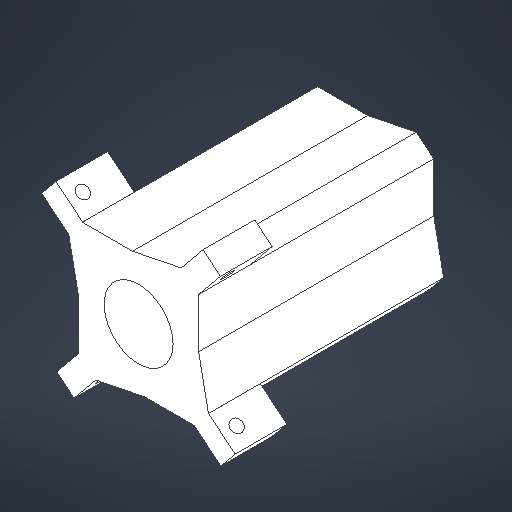
# Autodesk Inventor part: Lifter compartment
Saved by Autodesk Inventor 2026.1 (Build 301233020, 233B)
## iProperties
Created: 2025-11-27
Part Number: Lifter compartment
Material: Generic
Document SubType Name: Modeling
Designer: sarab
Density: 1 g/cm^3
Appearance: Default
Author: sarab
Autodesk Inventor part; units mm, degrees
ref_plane "YZ Plane" through (0, 0, 0) normal (1, 0, 0) x (0, 1, 0)
ref_plane "XZ Plane" through (0, 0, 0) normal (0, 1, 0) x (-1, 0, 0)
ref_plane "XY Plane" through (0, 0, 0) normal (0, 0, 1) x (1, 0, 0)
sketch "Sketch1" plane through (0, 0, 0) normal (0, 0, 1) x (1, 0, 0)
  circle A0 centre (-38.3507, 10.1677) radius 10.4
  line L0 (-51.23, -10.8726) -> (-51.1921, -10.9035)
  line L1 (-51.1921, -10.9035) -> (-36.539, -7.9419)
  line L2 (-36.539, -7.9419) -> (-21.5895, -7.9419)
  line L3 (-21.5895, -7.9419) -> (-13.5401, -14.5272)
  line L4 (-9.2136, -9.2389) -> (-13.5401, -14.5272)
  line L5 (-17.2631, -2.6536) -> (-9.2136, -9.2389)
  line L6 (-17.2631, -2.6536) -> (-17.2795, -2.6737)
  line L7 (-17.2795, -2.6737) -> (-20.2411, 11.9795)
  line L8 (-20.2411, 11.9795) -> (-20.2411, 26.9289)
  line L9 (-20.2411, 26.9289) -> (-13.6558, 34.9784)
  line L10 (-18.9241, 39.2883) -> (-13.6558, 34.9784)
  line L11 (-25.5094, 31.2389) -> (-18.9241, 39.2883)
  line L12 (-25.5094, 31.2389) -> (-40.1625, 28.2773)
  line L13 (-40.1625, 28.2773) -> (-55.3133, 28.2773)
  line L14 (-55.3133, 28.2773) -> (-55.2326, 28.3759)
  line L15 (-55.2326, 28.3759) -> (-63.282, 34.9612)
  line L16 (-67.592, 29.693) -> (-63.282, 34.9612)
  line L17 (-59.5426, 23.1077) -> (-67.592, 29.693)
  line L18 (-59.5426, 23.1077) -> (-59.4618, 23.2064)
  line L19 (-59.4618, 23.2064) -> (-56.4603, 8.3559)
  line L20 (-56.4603, 8.3559) -> (-56.4603, -6.5936)
  line L21 (-56.4603, -6.5936) -> (-63.0456, -14.643)
  line L22 (-57.8153, -18.922) -> (-63.0456, -14.643)
  line L23 (-51.23, -10.8726) -> (-57.8153, -18.922)
  circle A1 centre (-38.3507, 10.1677) radius 10.4
  line L24 (-51.23, -10.8726) -> (-51.1921, -10.9035)
  line L25 (-51.1921, -10.9035) -> (-36.539, -7.9419)
  line L26 (-36.539, -7.9419) -> (-21.5895, -7.9419)
  line L27 (-21.5895, -7.9419) -> (-13.5401, -14.5272)
  line L28 (-9.2136, -9.2389) -> (-13.5401, -14.5272)
  line L29 (-17.2631, -2.6536) -> (-9.2136, -9.2389)
  line L30 (-17.2631, -2.6536) -> (-17.2795, -2.6737)
  line L31 (-17.2795, -2.6737) -> (-20.2411, 11.9795)
  line L32 (-20.2411, 11.9795) -> (-20.2411, 26.9289)
  line L33 (-20.2411, 26.9289) -> (-13.6558, 34.9784)
  line L34 (-18.9241, 39.2883) -> (-13.6558, 34.9784)
  line L35 (-25.5094, 31.2389) -> (-18.9241, 39.2883)
  line L36 (-25.5094, 31.2389) -> (-40.1625, 28.2773)
  line L37 (-40.1625, 28.2773) -> (-55.3133, 28.2773)
  line L38 (-55.3133, 28.2773) -> (-55.2326, 28.3759)
  line L39 (-55.2326, 28.3759) -> (-63.282, 34.9612)
  line L40 (-67.592, 29.693) -> (-63.282, 34.9612)
  line L41 (-59.5426, 23.1077) -> (-67.592, 29.693)
  line L42 (-59.5426, 23.1077) -> (-59.4618, 23.2064)
  line L43 (-59.4618, 23.2064) -> (-56.4603, 8.3559)
  line L44 (-56.4603, 8.3559) -> (-56.4603, -6.5936)
  line L45 (-56.4603, -6.5936) -> (-63.0456, -14.643)
  line L46 (-57.8153, -18.922) -> (-63.0456, -14.643)
  line L47 (-51.23, -10.8726) -> (-57.8153, -18.922)
  point P0 (0, 0)
  constraints: 96 end point, 2 centre point
extrude "Extrusion1" add sketch "Sketch1" along normal blind 70.935
sketch "Sketch2" plane through (-59.5426, 23.1077, 0) normal (-0.6332026, -0.7739861, 0) x (0.7739861, -0.6332026, 0)
  line L0 (47.2215, 0) -> (47.2215, 55.335)
  line L1 (49.0358, 0) -> (49.0358, 70.935) projected
  line L2 (49.0358, 55.335) -> (60.717, 55.335)
  line L3 (60.717, 55.335) -> (60.717, 0)
  line L4 (60.717, 0) -> (49.0358, 0)
  constraints: 8 end point, 2 perpendicular, 1 horizontal, 1 point on line, 1 vertical
extrude "Extrusion2" cut sketch "Sketch2" against normal blind 70.935
sketch "Sketch3" plane through (-13.6558, 34.9784, 70.935) normal (0.7739861, -0.6332026, 0) x (0, 0, -1)
  line L0 (70.935, -21.9707) -> (70.935, -10.4) projected
  line L1 (70.935, -10.4) -> (15.6, -10.4)
  line L2 (70.935, -10.4) -> (0, -10.4) projected
  line L3 (15.6, -10.4) -> (15.6, 1.2922)
  line L4 (15.6, 1.2922) -> (70.935, 1.2922)
  line L5 (70.935, 1.2922) -> (70.935, -10.4)
  point P0 (70.935, -18.4258)
  constraints: 8 end point, 3 perpendicular, 1 point on line
extrude "Extrusion3" cut sketch "Sketch3" against normal blind 70.935
sketch "Sketch5" plane through (-63.282, 34.9612, 70.935) normal (0.6332026, 0.7739861, 0) x (0.7739861, -0.6332026, 0)
  line L0 (0, 70.935) -> (0, 0) projected
  line L1 (0, 70.935) -> (0, 15.6)
  line L2 (0, 15.6) -> (10.4, 15.6)
  line L3 (10.4, 70.935) -> (10.4, 0) projected
  line L4 (10.4, 15.6) -> (10.4, 70.935)
  line L5 (10.4, 70.935) -> (0, 70.935)
  point P0 (71.117, 70.935)
  point P1 (10.4, 15.6)
  constraints: 8 end point, 3 perpendicular, 1 point on line
extrude "Extrusion4" cut sketch "Sketch5" against normal blind 70.935
sketch "Sketch6" plane through (-63.0456, -14.643, 0) normal (-0.7739861, 0.6332026, 0) x (0, 0, 1)
  line L0 (0, 0) -> (0, 10.4) projected
  line L1 (0, 0) -> (55.335, 0)
  line L2 (0, 0) -> (70.935, 0) projected
  line L3 (55.335, 0) -> (55.335, 10.4601)
  line L4 (55.335, 10.4601) -> (0, 10.4601)
  line L5 (0, 10.4601) -> (0, 0)
  point P0 (0, 51.2542)
  constraints: 8 end point, 3 perpendicular, 1 point on line
extrude "Extrusion5" cut sketch "Sketch6" against normal blind 70.935
sketch "Sketch7" plane through (-13.6558, 34.9784, 70.935) normal (0.7739861, -0.6332026, 0) x (0, 0, -1)
  circle A0 centre (5.281, -5.0747) radius 1.841
  point P0 (70.935, -18.4258)
  constraints: 1 centre point
extrude "Extrusion6" cut sketch "Sketch7" against normal blind 70.935
sketch "Sketch8" plane through (-51.23, -10.8726, 70.935) normal (0.7739861, -0.6332026, 0) x (0, 0, -1)
  circle A0 centre (5.0992, -4.9107) radius 1.841
  point P0 (70.935, 40.8542)
  constraints: 1 centre point
extrude "Extrusion7" cut sketch "Sketch8" against normal blind 70.935
sketch "Sketch9" plane through (-13.5401, -14.5272, 55.335) normal (-0.6332026, -0.7739861, 0) x (0.7739861, -0.6332026, 0)
  circle A0 centre (-5.0967, 11.2282) radius 1.841
  circle A1 centre (-64.9486, 11.2282) radius 1.841
  point P0 (1.2811, -55.335)
  constraints: 2 centre point
extrude "Extrusion8" cut sketch "Sketch9" against normal blind 70.935
sketch "Sketch10" plane through (0, 0, 0) normal (0, 0, -1) x (-1, 0, 0)
  line L0 (22.3279, -5.5568) -> (19.104, -2.4278)
  line L1 (19.104, -2.4278) -> (23.2761, 11.2262)
  line L2 (23.2761, 11.2262) -> (23.2761, 26.1128)
  arc A0 (26.1681, 28.9573) -> (23.2761, 26.1128) centre (26.1211, 26.1128) ccw
  line L3 (26.1681, 28.9573) -> (40.1539, 26.1128)
  line L4 (40.1539, 26.1128) -> (53.066, 26.1128)
  line L5 (53.066, 26.1128) -> (56.4891, 22.7904)
  line L6 (50.9259, -7.8719) -> (54.7765, -5.1545)
  line L7 (54.7765, -5.1545) -> (54.7765, 8.6166)
  line L8 (54.7765, 8.6166) -> (56.4881, 23.4995)
  line L9 (51.7835, -7.2666) -> (36.3702, -5.5568)
  line L10 (36.3702, -5.5568) -> (22.3279, -5.5568)
  circle A1 centre (38.1545, 10.5282) radius 13.3756
  point P0 (0, 0)
  point P1 (56.4148, 22.8625)
  constraints: 22 end point, 2 centre point, 2 point on circle, 2 point on line, 2 vertical, 1 horizontal, 1 parallel, 1 perpendicular, 1 tangent
extrude "Extrusion9" cut sketch "Sketch10" against normal blind 64
body "Solid1"
